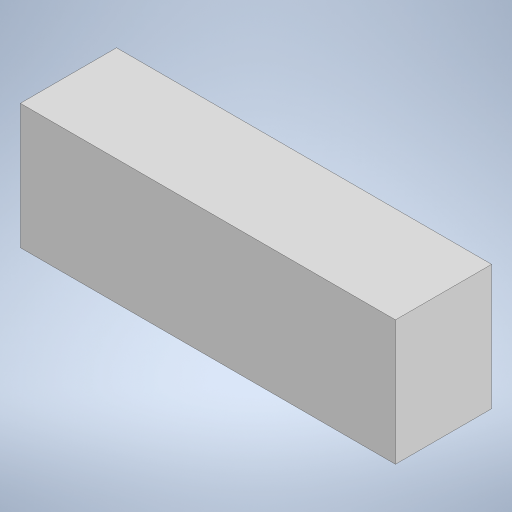
# Autodesk Inventor part: tlacitko
Saved by Autodesk Inventor 2023 (Build 270158000, 158)
## iProperties
Created: 2023-04-12
Part Number: tlacitko
Material: Všeobecné
Document SubType Name: Modeling
Designer: zak
Density: 1 g/cm^3
Appearance: Výchozí
Author: zak
Autodesk Inventor part; units mm, degrees
ref_plane "YZ Plane" through (0, 0, 0) normal (1, 0, 0) x (0, 1, 0)
ref_plane "XZ Plane" through (0, 0, 0) normal (0, 1, 0) x (-1, 0, 0)
ref_plane "XY Plane" through (0, 0, 0) normal (0, 0, 1) x (1, 0, 0)
sketch "Náčrt1" plane through (0, 0, 0) normal (0, 0, 1) x (1, 0, 0)
  line L0 (-9.75, -3.25) -> (9.75, -3.25)
  line L1 (9.75, -3.25) -> (9.75, 3.25)
  line L2 (9.75, 3.25) -> (-9.75, 3.25)
  line L3 (-9.75, 3.25) -> (-9.75, -3.25)
  line L4 (-9.75, -3.25) -> (9.75, 3.25) construction
  line L5 (9.75, -3.25) -> (-9.75, 3.25) construction
  point P0 (0, 0)
  dimension "d0" = 19.5
  dimension "d1" = 6.5
  constraints: 12 end point, 2 midpoint, 2 parallel, 1 horizontal, 1 perpendicular
  measures "d0" distance of L2.end L1.end
  measures "d1" distance of L1.end L0.end
extrude "Vysunutí1" add sketch "Náčrt1" along normal blind 5
